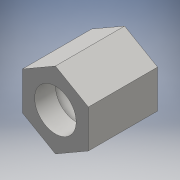
# Autodesk Inventor part: M8x6 Pipe Nut
Saved by Autodesk Inventor 2016 (Build 200138000, 138)
## iProperties
Created: 2016-12-04
Part Number: M8x6 Pipe Nut
Material: Generic
Document SubType Name: Modeling
Designer: Muhammad
Density: 1 g/cm^3
Appearance: Default
Author: Muhammad
Autodesk Inventor part; units mm, degrees
ref_plane "YZ Plane" through (0, 0, 0) normal (1, 0, 0) x (0, 1, 0)
ref_plane "XZ Plane" through (0, 0, 0) normal (0, 1, 0) x (-1, 0, 0)
ref_plane "XY Plane" through (0, 0, 0) normal (0, 0, 1) x (1, 0, 0)
sketch "Sketch1" plane through (0, 0, 0) normal (0, 1, 0) x (-1, 0, 0)
  line L0 (0, 0) -> (0, -5.5)
  line L1 (0, -5.5) -> (-4.7631, -2.75)
  line L2 (-4.7631, -2.75) -> (-4.7631, 2.75)
  line L3 (-4.7631, 2.75) -> (0, 5.5)
  line L4 (0, 5.5) -> (4.7631, 2.75)
  line L5 (4.7631, 2.75) -> (4.7631, -2.75)
  line L6 (4.7631, -2.75) -> (0, -5.5)
  dimension "d0" = 5.5
  constraints: 14 end point, 1 coincident, 1 vertical, 13 other
  measures "d0" distance of L0.start L0.end
extrude "Extrusion1" add sketch "Sketch1" along normal blind 10
sketch "Sketch2" plane through (0, 10, 0) normal (0, 1, 0) x (1, 0, 0)
  circle A0 centre (0, 0) radius 4
  dimension "d3" = 8
  constraints: 1 centre point, 1 coincident
  measures "d3" diameter of A0
hole "Hole1" at (0, 10, 0) direction (0, -1, 0) diameter 6 depth 10 tip angle 118 counterbore diameter 8 counterbore depth 7
body "Solid1"
